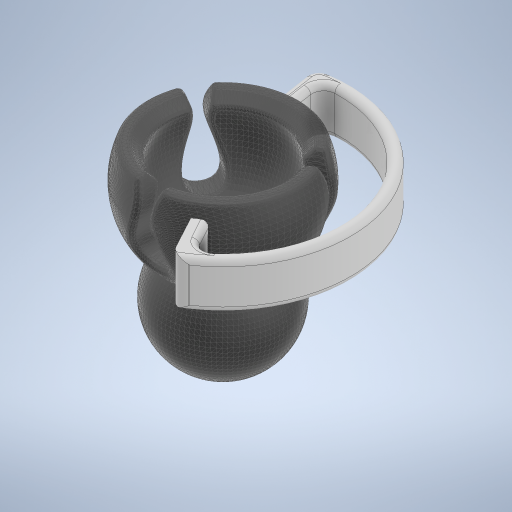
# Autodesk Inventor part: New_12_BallSocket_Joint
Saved by Autodesk Inventor 2024.2 (Build 282272000, 272)
## iProperties
Created: 2025-05-26
Part Number: New_12_BallSocket_Joint
Material: Všeobecné
Document SubType Name: Modeling
Designer: Elite
Density: 1 g/cm^3
Appearance: Výchozí
Author: Elite
Autodesk Inventor part; units mm, degrees
ref_plane "YZ Plane" through (0, 0, 0) normal (1, 0, 0) x (0, 1, 0)
ref_plane "XZ Plane" through (0, 0, 0) normal (0, 1, 0) x (-1, 0, 0)
ref_plane "Pracovní rovina1" through (0, 0, 10) normal (0, 0, 1) x (1, 0, 0)
sketch "Náčrt1" plane through (0, 0, 10) normal (0, 0, 1) x (1, 0, 0)
  circle A0 centre (-0.00001, -2.065606) radius 2.26126
  circle A1 centre (-0.00001, -2.065606) radius 7.021943
  line L0 (3.33745, -8.243716) -> (5.23861, -11.763032)
  arc A2 (3.123739, -7.848107) -> (4.055891, -7.237143) centre (-0.00001, -2.065606) ccw
  line L1 (3.33745, -8.243716) -> (3.123739, -7.848107)
  line L2 (4.290615, -7.624222) -> (4.055891, -7.237143)
  arc A3 (5.23861, -11.763032) -> (-2.733425, 8.612019) centre (-0.00001, -2.065606) ccw
  line L3 (5.23861, -11.763032) -> (6.220522, -11.164408)
  line L4 (6.220522, -11.164408) -> (4.055891, -7.237143)
  arc A4 (4.76332, -10.883203) -> (-1.460281, 7.84938) centre (-0.00001, -2.065606) ccw
  line L5 (-1.023159, 4.881397) -> (-1.605989, 8.838708)
  arc A5 (-0.957643, 4.436553) -> (-2.042541, 4.181249) centre (-0.00001, -2.065606) ccw
  line L6 (-1.023159, 4.881397) -> (-0.957643, 4.436553)
  line L7 (-2.130721, 4.625265) -> (-2.042541, 4.181249)
  line L8 (-1.605989, 8.838708) -> (-2.733425, 8.612019)
  line L9 (-2.733425, 8.612019) -> (-2.042541, 4.181249)
  point P0 (0, 0)
  point P1 (5.735356, -10.284177)
  point P2 (4.275608, -7.635774)
  dimension "d2" = 4
  dimension "d7" = 1.15
  dimension "d8" = 1
  dimension "d11" = 160
  constraints: 20 end point, 11 point on circle, 5 centre point, 4 coincident, 2 point on line, 14 other
  measures "d2" distance of L0.start L0.end
  measures "d7" distance of L0.end L3.end
  measures "d8" radial gap between concentric circles of A3 A4
extrude "Vysunutí1" add sketch "Náčrt1" along normal mid plane 4 contours L6 A5 L9 A1 | A1 L9 L8 L5 | L5 A3 L4 A4 | L4 A4 L0 A1 | A1 L1 A2 L4 | L4 L3 L0 A4
fillet "Zaoblení2" radius 1 4 edges at (-2.7334, 8.612, 10) (-1.4603, 7.8494, 10) (5.2386, -11.763, 10) (5.7354, -10.2842, 10)
fillet "Zaoblení3" radius 0.5 18 edges at (10.2642, 1.9504, 8) (10.2642, 1.9504, 12) (-2.4182, 8.3922, 8) (-1.7005, 8.8197, 8) (-2.3142, 5.9238, 8) (9.2906, 1.6926, 8) (5.8748, -9.7528, 8) (4.6104, -8.2433, 8) (-1.1321, 5.6208, 8) (-1.0854, 7.5909, 8) (-1.7005, 8.8197, 12) (-2.3142, 5.9238, 12) (-2.4182, 8.3922, 12) (-1.1321, 5.6208, 12) (9.2906, 1.6926, 12) (5.8748, -9.7528, 12) (4.6104, -8.2433, 12) (-1.0854, 7.5909, 12)
